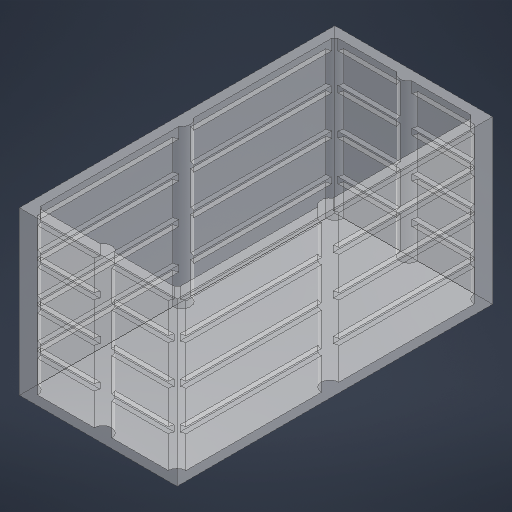
# Autodesk Inventor part: Part7
Saved by Autodesk Inventor 2026 (Build 300175000, 175)
## iProperties
Created: 2026-02-26
Part Number: Part7
Material: PET Plastic
Document SubType Name: Modeling
Designer: Usuario2
Density: 1.541 g/cm^3
Appearance: Polycarbonate - Clear
Mass: 58.4824 g
Surface Area: 443.743 cm^2
Volume: 37.9509 cm^3
Author: Usuario2
Autodesk Inventor part; units mm, degrees
ref_plane "YZ Plane" through (0, 0, 0) normal (1, 0, 0) x (0, 1, 0)
ref_plane "XZ Plane" through (0, 0, 0) normal (0, 1, 0) x (-1, 0, 0)
sketch "Sketch1" plane through (0, 0, 0) normal (0, 1, 0) x (-1, 0, 0)
  line L0 (25.4, 50.8) -> (-25.4, 50.8)
  line L1 (-25.4, 50.8) -> (-25.4, -50.8)
  line L2 (-25.4, -50.8) -> (25.4, -50.8)
  line L3 (25.4, -50.8) -> (25.4, 50.8)
  line L4 (25.4, 50.8) -> (-25.4, -50.8) construction
  line L5 (-25.4, 50.8) -> (25.4, -50.8) construction
  point P0 (0, 0)
  dimension "d0" = 50.8
  dimension "d1" = 101.6
  constraints: 12 end point, 2 midpoint, 2 parallel, 1 horizontal, 1 perpendicular
  measures "d0" distance of L2.end L1.end
  measures "d1" distance of L1.end L0.end
extrude "Extrusion1" add sketch "Sketch1" along normal blind 1.5
sketch "Sketch2" plane through (0, 1.5, 0) normal (0, 1, 0) x (1, 0, 0)
  line L0 (-25.4, 50.8) -> (25.4, 50.8)
  line L1 (25.4, 50.8) -> (25.4, -50.8)
  line L2 (25.4, -50.8) -> (-25.4, -50.8)
  line L3 (-25.4, -50.8) -> (-25.4, 50.8)
  line L4 (-25.4, 50.8) -> (25.4, -50.8) construction
  line L5 (25.4, 50.8) -> (-25.4, -50.8) construction
  line L6 (25.4, -50.8) -> (23.9, -50.8)
  line L7 (23.9, -50.8) -> (23.9, -49.3)
  line L8 (23.9, -49.3) -> (25.4, -49.3)
  line L9 (25.4, -49.3) -> (25.4, -50.8)
  line L10 (-25.4, 50.8) -> (-23.9, 50.8)
  line L11 (-23.9, 50.8) -> (-23.9, 49.3)
  line L12 (-23.9, 49.3) -> (-25.4, 49.3)
  line L13 (-25.4, 49.3) -> (-25.4, 50.8)
  line L14 (-23.9, 49.3) -> (23.9, 49.3)
  line L15 (23.9, 49.3) -> (23.9, -49.3)
  line L16 (23.9, -49.3) -> (-23.9, -49.3)
  line L17 (-23.9, -49.3) -> (-23.9, 49.3)
  point P0 (0, 0)
  dimension "d4" = 50.8
  dimension "d5" = 101.6
  dimension "d6" = 1.5
  dimension "d7" = 1.5
  dimension "d8" = 1.5
  dimension "d9" = 1.5
  constraints: 36 end point, 8 parallel, 4 horizontal, 4 perpendicular, 2 midpoint
  measures "d4" distance of L1.end L2.end
  measures "d5" distance of L0.end L1.end
  measures "d6" distance of L7.end L8.end
  measures "d7" distance of L6.end L7.end
  measures "d8" distance of L11.end L12.end
  measures "d9" distance of L10.end L11.end
extrude "Extrusion2" add sketch "Sketch2" along normal blind 50.8 contours L0 L11 L12 L3 | L0 L1 L8 L15 L14 L11 | L12 L17 L16 L7 L2 L3 | L1 L2 L7 L8
sketch "Sketch3" plane through (0, 1.5, 0) normal (0, 1, 0) x (1, 0, 0)
  line L0 (-23.9, -49.3) -> (-23.9, 49.3) projected
  line L1 (23.9, -49.3) -> (-23.9, -49.3)
  line L2 (-23.9, -49.3) -> (-23.9, 49.3)
  line L3 (-23.9, 49.3) -> (23.9, 49.3)
  line L4 (23.9, 49.3) -> (23.9, -49.3)
  line L5 (23.9, -49.3) -> (-23.9, 49.3) construction
  line L6 (-23.9, -49.3) -> (23.9, 49.3) construction
  line L7 (-23.9, -49.3) -> (-21.9, -49.3)
  line L8 (-21.9, -49.3) -> (-21.9, -47.3)
  line L9 (-21.9, -47.3) -> (-23.9, -47.3)
  line L10 (-23.9, -47.3) -> (-23.9, -49.3)
  circle A0 centre (-23.9, -49.3) radius 2.8284
  circle A1 centre (-23.9, -0.024) radius 2.8284
  circle A2 centre (-23.9, 49.252) radius 2.8284
  circle A3 centre (-0.024, -49.3) radius 2.8284
  circle A4 centre (-0.024, -0.024) radius 2.8284
  circle A5 centre (-0.024, 49.252) radius 2.8284
  circle A6 centre (23.852, -49.3) radius 2.8284
  circle A7 centre (23.852, -0.024) radius 2.8284
  circle A8 centre (23.852, 49.252) radius 2.8284
  point P0 (0, 0)
  point P1 (-21.0716, -49.3)
  point P2 (-23.9, -46.4716)
  point P3 (-21.9, 1.976)
  point P4 (-21.9, 51.252)
  point P5 (1.976, -47.3)
  point P6 (1.976, 1.976)
  point P7 (1.976, 51.252)
  point P8 (25.852, -47.3)
  point P9 (25.852, 1.976)
  point P10 (25.852, 51.252)
  point P11 (-23.9, 2.8044)
  point P12 (-23.9, -2.8524)
  point P13 (-21.072, 49.3)
  point P14 (-23.9, 46.4236)
  point P15 (-2.852, 49.3)
  point P16 (2.804, 49.3)
  point P17 (21.024, 49.3)
  point P18 (23.9, 46.424)
  point P19 (23.9, -2.852)
  point P20 (23.9, 2.804)
  point P21 (23.9, -46.472)
  point P22 (21.0236, -49.3)
  point P23 (-2.8524, -49.3)
  point P24 (2.8044, -49.3)
  dimension "d12" = 2
  dimension "d13" = 2
  dimension "d18" = 49.276
  dimension "d21" = 23.876
  constraints: 20 end point, 9 horizontal, 4 parallel, 3 vertical, 2 midpoint, 2 perpendicular, 1 coincident, 43 other
  measures "d12" distance of L9.end L8.end
  measures "d13" distance of L8.end L7.end
  measures "d18" distance of point (-23.9, -49.3) point (-23.9, -0.024)
  measures "d21" distance of point (-23.9, -49.3) point (-0.024, -49.3)
extrude "Extrusion3" add sketch "Sketch3" along normal blind 50.8 contours L0 L9 L8 L1 | L0 A0 L9 | L8 A0 L1 | L0 A1 | A3 L1 | L0 L3 A2 | A6 L4 L1 | L3 A5 | A7 L4 | L3 L4 A8 picked at (-22.9572, -0.024) picked at (0.6817, -48.6748) picked at (-23.6902, 47.406) picked at (22.0065, -49.088) picked at (-0.1462, 48.3492) picked at (22.085, 0.0683) picked at (22.5434, 47.9434)
ref_plane "Work Plane1" through (0, 12.7, 0) normal (0, -1, 0) x (1, 0, 0)
sketch "Sketch4" plane through (0, 12.7, 0) normal (0, -1, 0) x (1, 0, 0)
  line L0 (-25.4, 50.8) -> (25.4, 50.8)
  line L1 (25.4, 50.8) -> (25.4, -50.8)
  line L2 (25.4, -50.8) -> (-25.4, -50.8)
  line L3 (-25.4, -50.8) -> (-25.4, 50.8)
  line L4 (-25.4, 50.8) -> (25.4, -50.8) construction
  line L5 (25.4, 50.8) -> (-25.4, -50.8) construction
  line L6 (-25.4, -50.8) -> (-22.4, -50.8)
  line L7 (-22.4, -50.8) -> (-22.4, -47.8)
  line L8 (-22.4, -47.8) -> (-25.4, -47.8)
  line L9 (-25.4, -47.8) -> (-25.4, -50.8)
  line L10 (25.4, 50.8) -> (22.4, 50.8)
  line L11 (22.4, 50.8) -> (22.4, 47.8)
  line L12 (22.4, 47.8) -> (25.4, 47.8)
  line L13 (25.4, 47.8) -> (25.4, 50.8)
  line L14 (22.4, 47.8) -> (-22.4, 47.8)
  line L15 (-22.4, 47.8) -> (-22.4, -47.8)
  line L16 (-22.4, -47.8) -> (22.4, -47.8)
  line L17 (22.4, -47.8) -> (22.4, 47.8)
  point P0 (0, 0)
  dimension "d25" = 50.8
  dimension "d26" = 101.6
  dimension "d27" = 3
  dimension "d28" = 3
  dimension "d29" = 3
  dimension "d30" = 3
  constraints: 36 end point, 8 parallel, 4 horizontal, 4 perpendicular, 2 midpoint
  measures "d25" distance of L1.end L2.end
  measures "d26" distance of L0.end L1.end
  measures "d27" distance of L8.end L7.end
  measures "d28" distance of L7.end L6.end
  measures "d29" distance of L12.end L11.end
  measures "d30" distance of L11.end L10.end
extrude "Extrusion4" add sketch "Sketch4" along normal mid plane 2 contours L0 L11 L14 L15 L8 L3 | L0 L1 L12 L11 | L8 L7 L2 L3 | L12 L1 L2 L7 L16 L17
ref_plane "Work Plane2" through (0, 25.4, 0) normal (0, -1, 0) x (1, 0, 0)
sketch "Sketch5" plane through (0, 25.4, 0) normal (0, -1, 0) x (1, 0, 0)
  line L0 (25.4, -50.8) -> (-25.4, -50.8) projected
  line L1 (-25.4, 50.8) -> (25.4, 50.8)
  line L2 (25.4, 50.8) -> (25.4, -50.8)
  line L3 (25.4, -50.8) -> (-25.4, -50.8)
  line L4 (-25.4, -50.8) -> (-25.4, 50.8)
  line L5 (-25.4, 50.8) -> (25.4, -50.8) construction
  line L6 (25.4, 50.8) -> (-25.4, -50.8) construction
  line L7 (-22.4, -47.8) -> (22.4, -47.8)
  line L8 (22.4, -47.8) -> (22.4, 47.8)
  line L9 (22.4, 47.8) -> (-22.4, 47.8)
  line L10 (-22.4, 47.8) -> (-22.4, -47.8)
  line L11 (-22.4, -47.8) -> (22.4, 47.8) construction
  line L12 (22.4, -47.8) -> (-22.4, 47.8) construction
  point P0 (0, 0)
  dimension "d34" = 50.8
  dimension "d35" = 101.6
  dimension "d36" = 44.8
  dimension "d37" = 95.6
  constraints: 24 end point, 4 midpoint, 4 parallel, 2 horizontal, 2 perpendicular
  measures "d34" distance of L0.start L3.end
  measures "d35" distance of L1.end L0.start
  measures "d36" distance of L9.end L8.end
  measures "d37" distance of L8.end L7.end
extrude "Extrusion5" add sketch "Sketch5" along normal mid plane 2
ref_plane "Work Plane3" through (0, 38.1, 0) normal (0, -1, 0) x (1, 0, 0)
sketch "Sketch6" plane through (0, 38.1, 0) normal (0, -1, 0) x (1, 0, 0)
  line L0 (25.4, 50.8) -> (-25.4, 50.8)
  line L1 (-25.4, 50.8) -> (-25.4, -50.8)
  line L2 (-25.4, -50.8) -> (25.4, -50.8)
  line L3 (25.4, -50.8) -> (25.4, 50.8)
  line L4 (25.4, 50.8) -> (-25.4, -50.8) construction
  line L5 (-25.4, 50.8) -> (25.4, -50.8) construction
  line L6 (-22.4, 47.8) -> (22.4, 47.8)
  line L7 (22.4, 47.8) -> (22.4, -47.8)
  line L8 (22.4, -47.8) -> (-22.4, -47.8)
  line L9 (-22.4, -47.8) -> (-22.4, 47.8)
  line L10 (-22.4, 47.8) -> (22.4, -47.8) construction
  line L11 (22.4, 47.8) -> (-22.4, -47.8) construction
  point P0 (0, 0)
  dimension "d41" = 50.8
  dimension "d42" = 101.6
  dimension "d43" = 44.8
  dimension "d44" = 95.6
  constraints: 24 end point, 4 midpoint, 4 parallel, 2 horizontal, 2 perpendicular
  measures "d41" distance of L2.end L1.end
  measures "d42" distance of L1.end L0.end
  measures "d43" distance of L7.end L8.end
  measures "d44" distance of L6.end L7.end
extrude "Extrusion6" add sketch "Sketch6" along normal mid plane 2
ref_plane "Work Plane4" through (0, 50.8, 0) normal (0, -1, 0) x (1, 0, 0)
sketch "Sketch7" plane through (0, 50.8, 0) normal (0, -1, 0) x (1, 0, 0)
  line L0 (25.4, 50.8) -> (25.4, -50.8) projected
  line L1 (-25.4, 50.8) -> (25.4, 50.8)
  line L2 (25.4, 50.8) -> (25.4, -50.8)
  line L3 (25.4, -50.8) -> (-25.4, -50.8)
  line L4 (-25.4, -50.8) -> (-25.4, 50.8)
  line L5 (-25.4, 50.8) -> (25.4, -50.8) construction
  line L6 (25.4, 50.8) -> (-25.4, -50.8) construction
  line L7 (-22.4, 47.8) -> (22.4, 47.8)
  line L8 (22.4, 47.8) -> (22.4, -47.8)
  line L9 (22.4, -47.8) -> (-22.4, -47.8)
  line L10 (-22.4, -47.8) -> (-22.4, 47.8)
  line L11 (-22.4, 47.8) -> (22.4, -47.8) construction
  line L12 (22.4, 47.8) -> (-22.4, -47.8) construction
  point P0 (0, 0)
  dimension "d48" = 50.8
  dimension "d49" = 101.6
  dimension "d50" = 44.8
  dimension "d51" = 95.6
  constraints: 24 end point, 4 midpoint, 4 parallel, 2 horizontal, 2 perpendicular
  measures "d48" distance of L0.end L3.end
  measures "d49" distance of L1.end L0.end
  measures "d50" distance of L8.end L9.end
  measures "d51" distance of L7.end L8.end
extrude "Extrusion7" add sketch "Sketch7" along normal blind 2 and the other way blind 1.5
body "Solid1"
